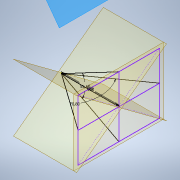
# Autodesk Inventor part: cameraFOV
Saved by Autodesk Inventor 2020 (Build 240168000, 168)
## iProperties
Created: 2022-10-12
Part Number: cameraFOV
Material: Типовые
Document SubType Name: Modeling
Designer: akapu
Density: 1 g/cm^3
Appearance: По умолчанию
Author: akapu
Autodesk Inventor part; units mm, degrees
ref_plane "XZ Plane" through (0, 0, 0) normal (0, 1, 0) x (-1, 0, 0)
ref_plane "XY Plane" through (0, 0, 0) normal (0, 0, 1) x (1, 0, 0)
sketch "Эскиз1" plane through (0, 0, 0) normal (0, 0, 1) x (1, 0, 0)
  line L0 (0, 0) -> (100, 0)
  line L1 (0, 0) -> (100, -52.724)
  line L2 (0, 0) -> (100, 52.724)
  line L3 (100, -52.724) -> (100, 52.724)
  line L4 (100, 52.724) -> (100, -52.724)
  line L5 (100, -52.724) -> (0, -52.724)
  line L6 (0, -52.724) -> (0, 52.724)
  line L7 (0, 52.724) -> (100, 52.724)
  dimension "d0" = 100
  dimension "d2" = 55.6
  constraints: 16 end point, 2 parallel, 2 vertical, 1 horizontal, 1 perpendicular, 1 symmetric about line
  measures "d0" distance of L0.start L0.end
  measures "d2" angle of L2 L1
sketch "Эскиз2" plane through (0, 0, 0) normal (0, 1, 0) x (-1, 0, 0)
  line L0 (0, 0) -> (-100, 0)
  line L1 (0, 0) -> (-100, -71.0663)
  line L2 (0, 0) -> (-100, 71.0663)
  line L3 (-100, -71.0663) -> (-100, 71.0663)
  dimension "d3" = 100
  dimension "d5" = 70.8
  constraints: 8 end point, 1 horizontal, 1 symmetric about line, 1 vertical
  measures "d3" distance of L0.start L0.end
  measures "d5" angle of L2 L1
ref_plane "РабПлоскость1" through (100, 0, 0) normal (1, 0, 0) x (0, 1, 0)
sketch "Эскиз3" plane through (100, 0, 0) normal (1, 0, 0) x (0, 1, 0)
  line L0 (0, 0) -> (0, -71.0663) projected
  line L1 (0, -71.0663) -> (0, 71.0663) projected
  line L2 (-52.724, 0) -> (52.724, 0) projected
  line L3 (-52.724, 71.0663) -> (52.724, 71.0663)
  line L4 (52.724, 71.0663) -> (52.724, -71.0663)
  line L5 (52.724, -71.0663) -> (-52.724, -71.0663)
  line L6 (-52.724, -71.0663) -> (-52.724, 71.0663)
  line L7 (-52.724, 71.0663) -> (52.724, -71.0663) construction
  line L8 (52.724, 71.0663) -> (-52.724, -71.0663) construction
  constraints: 12 end point, 3 parallel, 2 midpoint, 1 perpendicular
extrude "Выдавливание1" add sketch "Эскиз2" along normal mid plane 105.448
extrude "Выдавливание2" cut sketch "Эскиз1" along normal mid plane 142.133 contours L6 L7 L2 | L1 L5 L6
ref_plane "РабПлоскость4" through (100, 52.724, -71.0663) normal (0, -0.8031, -0.5958) x (0, -0.5958, 0.8031)
ref_plane "РабПлоскость5" through (100, 52.724, 71.0663) normal (0, 0.8031, -0.5958) x (0, -0.5958, -0.8031)
sketch "Эскиз7" plane through (100, 52.724, -71.0663) normal (0, -0.8031, -0.5958) x (0, -0.5958, 0.8031)
  line L0 (62.8289, 0) -> (176.9773, 0) projected
  line L1 (176.9773, 0) -> (88.4886, 100)
  line L2 (88.4886, 100) -> (0, 0) projected
  line L3 (88.4886, 100) -> (0, 0)
  line L4 (0, 0) -> (176.9773, 0)
  constraints: 6 end point, 1 collinear
sketch "Эскиз8" plane through (100, 52.724, 71.0663) normal (0, 0.8031, -0.5958) x (0, -0.5958, -0.8031)
  line L0 (62.8289, 0) -> (0, 0) projected
  line L1 (176.9772, 0) -> (88.4886, 100) projected
  line L2 (0, 0) -> (88.4886, 100)
  line L3 (88.4886, 100) -> (176.9772, 0)
  line L4 (114.1484, 0) -> (176.9773, 0) projected
  line L5 (176.9772, 0) -> (0, 0)
  line L6 (88.4886, 100) -> (88.4886, 0)
  line L7 (176.9773, 0) -> (62.8289, 0) projected
  constraints: 8 end point, 1 collinear, 1 perpendicular, 1 point on line
